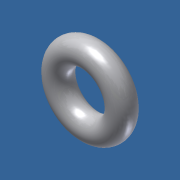
# Autodesk Inventor part: 1163N104
Saved by Autodesk Inventor 2015 SP1 (Build 190203100, 203)
## iProperties
Created: 2012-08-06
Part Number: 1163N104
Material: Generic
Vendor: MCMASTER
Document SubType Name: Modeling
Designer: NEGRASHOVI
Density: 1 g/cm^3
Mass: 0.0296144 g
Surface Area: 0.746188 cm^2
Volume: 0.0296144 cm^3
Description: VITON CLEAN ROOM O-RING DASH # 006
Project: COMMON
Appearance: Default
RuleStatus: InUse
AfterDocSave0: file://Part Number Cleaner
LAB/DEPT: COMMON
REQUESTING SCIENTIST: COMMON
SURFACE ROUGHNESS: N/A
DESIGN DEPARTMENT: HHMI: JRC - ID&F
SPECIAL FINISH: NONE
ALTERED ITEM PART NUMBER: N/A
ALTERED ITEM VENDOR: N/A
ALTERED ITEM DESCRIPTION: N/A
Revision Number: -
Autodesk Inventor part; units mm, degrees
ref_plane "YZ Plane" through (0, 0, 0) normal (1, 0, 0) x (0, 1, 0)
ref_plane "XZ Plane" through (0, 0, 0) normal (0, 1, 0) x (-1, 0, 0)
ref_plane "XY Plane" through (0, 0, 0) normal (0, 0, 1) x (1, 0, 0)
sketch "Sketch1" plane through (0, 0, 0) normal (0, 0, 1) x (1, 0, 0)
  circle A0 centre (0, 0) radius 2.3368
  dimension "d0" = 4.6736
  constraints: 1 centre point, 1 coincident
  measures "d0" diameter of A0
sketch "Sketch2" plane through (0, 0, 0) normal (1, 0, 0) x (0, 1, 0)
  line L0 (2.3368, 0) -> (-2.3368, 0) projected
  circle A0 centre (-2.3368, 0) radius 0.889
  point P0 (0, 0)
  dimension "d1" = 1.778
  constraints: 1 centre point, 1 coincident
  measures "d1" diameter of A0
sweep "Sweep1" add profiles "Sketch2" path "Sketch1"
body "Solid1"
